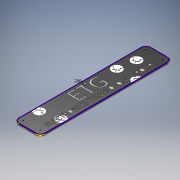
# Autodesk Inventor part: EtgSignModV5Texture2
Saved by Autodesk Inventor 2019 (Build 230136000, 136)
## iProperties
Created: 2018-10-30
Part Number: EtgSignModV5Texture2
Material: Generic
Document SubType Name: Modeling
Designer: Administrator
Density: 1 g/cm^3
Appearance: Default
Author: Administrator
Autodesk Inventor part; units mm, degrees
ref_plane "YZ Plane" through (0, 0, 0) normal (1, 0, 0) x (0, 1, 0)
ref_plane "XZ Plane" through (0, 0, 0) normal (0, 1, 0) x (-1, 0, 0)
ref_plane "XY Plane" through (0, 0, 0) normal (0, 0, 1) x (1, 0, 0)
sketch "Sketch1" plane through (0, 0, 0) normal (0, 1, 0) x (-1, 0, 0)
  line L0 (53.975, 0) -> (250.825, 0)
  line L1 (304.8, -53.975) -> (304.8, -1470.025)
  line L2 (250.825, -1524) -> (53.975, -1524)
  line L3 (0, -1470.025) -> (0, -53.975)
  circle A0 centre (263.525, -41.275) radius 5.5563
  circle A1 centre (263.525, -762) radius 5.5563
  circle A2 centre (263.525, -1482.725) radius 5.5563
  circle A3 centre (41.275, -41.275) radius 5.5563
  circle A4 centre (41.275, -762) radius 5.5563
  circle A5 centre (41.275, -1482.725) radius 5.5563
  arc A6 (304.8, -53.975) -> (250.825, 0) centre (250.825, -53.975) ccw
  arc A7 (0, -1470.025) -> (53.975, -1524) centre (53.975, -1470.025) ccw
  arc A8 (250.825, -1524) -> (304.8, -1470.025) centre (250.825, -1470.025) ccw
  arc A9 (53.975, 0) -> (0, -53.975) centre (53.975, -53.975) ccw
  point P0 (0, 0)
  point P1 (304.8, -1524)
  point P2 (0, -1524)
  dimension "d0" = 304.8
  dimension "d1" = 1524
  dimension "d2" = 11.1125
  dimension "d5" = 720.725
  dimension "d8" = 222.25
  dimension "d11" = 41.275
  dimension "d12" = 41.275
  dimension "d13" = 53.975
  constraints: 10 centre point, 8 end point, 8 point on circle, 8 tangent, 6 point on line, 3 equal radius, 2 horizontal, 2 parallel, 1 perpendicular, 1 vertical, 10 other
  measures "d0" distance of point (304.8, -1524) point (0, -1524)
  measures "d1" distance between parallel lines of L2 L0
  measures "d2" diameter of A0
  measures "d5" distance of A0.centre A1.centre
  measures "d8" distance of A0.centre A3.centre
  measures "d11" distance from line of L0 A0.centre
  measures "d12" distance from line of L1 A0.centre
  measures "d13" radius of A6
extrude "Extrusion1" add sketch "Sketch1" along normal blind 22.225
ref_plane "Work Plane3" through (0, 17.4625, 0) normal (0, 1, 0) x (1, 0, 0)
sketch "Sketch2" plane through (0, 17.4625, 0) normal (0, 1, 0) x (1, 0, 0)
  circle A0 centre (-41.275, 1482.725) radius 5.5562 projected
  circle A1 centre (-41.275, 762) radius 5.5562 projected
  circle A2 centre (-41.275, 41.275) radius 5.5562 projected
  circle A3 centre (-263.525, 1482.725) radius 5.5562 projected
  circle A4 centre (-263.525, 762) radius 5.5562 projected
  circle A5 centre (-263.525, 41.275) radius 5.5562 projected
  line L0 (-250.825, 0) -> (-53.975, 0) projected
  arc A6 (-53.975, 0) -> (0, 53.975) centre (-53.975, 53.975) ccw projected
  line L1 (0, 53.975) -> (0, 1470.025) projected
  arc A7 (0, 1470.025) -> (-53.975, 1524) centre (-53.975, 1470.025) ccw projected
  line L2 (-53.975, 1524) -> (-250.825, 1524) projected
  arc A8 (-250.825, 1524) -> (-304.8, 1470.025) centre (-250.825, 1470.025) ccw projected
  line L3 (-304.8, 1470.025) -> (-304.8, 53.975) projected
  arc A9 (-304.8, 53.975) -> (-250.825, 0) centre (-250.825, 53.975) ccw projected
  line L4 (0, 53.975) -> (0, 1470.025)
  arc A10 (-250.825, 1524) -> (-304.8, 1470.025) centre (-250.825, 1470.025) ccw projected
  line L5 (-53.975, 1524) -> (-250.825, 1524)
  line L6 (-304.8, 1470.025) -> (-304.8, 53.975) projected
  line L7 (-304.8, 1470.025) -> (-304.8, 53.975)
  line L8 (-250.825, 0) -> (-53.975, 0)
  point P0 (0, 0)
  constraints: 8 end point, 2 horizontal, 2 vertical, 1 tangent
ref_plane "Work Plane4" through (0, 4.7625, 0) normal (0, -1, 0) x (1, 0, 0)
sketch "Sketch3" plane through (0, 4.7625, 0) normal (0, -1, 0) x (1, 0, 0)
  circle A0 centre (-41.275, -1482.725) radius 5.5562 projected
  circle A1 centre (-41.275, -762) radius 5.5562 projected
  circle A2 centre (-41.275, -41.275) radius 5.5562 projected
  circle A3 centre (-263.525, -1482.725) radius 5.5562 projected
  circle A4 centre (-263.525, -762) radius 5.5562 projected
  circle A5 centre (-263.525, -41.275) radius 5.5562 projected
  line L0 (-250.825, 0) -> (-53.975, 0) projected
  arc A6 (0, -53.975) -> (-53.975, 0) centre (-53.975, -53.975) ccw projected
  line L1 (0, -53.975) -> (0, -1470.025) projected
  arc A7 (-53.975, -1524) -> (0, -1470.025) centre (-53.975, -1470.025) ccw projected
  line L2 (-53.975, -1524) -> (-250.825, -1524) projected
  arc A8 (-304.8, -1470.025) -> (-250.825, -1524) centre (-250.825, -1470.025) ccw projected
  line L3 (-304.8, -1470.025) -> (-304.8, -53.975) projected
  arc A9 (-250.825, 0) -> (-304.8, -53.975) centre (-250.825, -53.975) ccw projected
  line L4 (-299.72, -53.975) -> (-299.72, -1470.025)
  arc A10 (-299.72, -1470.025) -> (-250.825, -1518.92) centre (-250.825, -1470.025) ccw
  line L5 (-250.825, -1518.92) -> (-53.975, -1518.92)
  arc A11 (-53.975, -1518.92) -> (-5.08, -1470.025) centre (-53.975, -1470.025) ccw
  line L6 (-5.08, -1470.025) -> (-5.08, -53.975)
  arc A12 (-5.08, -53.975) -> (-53.975, -5.08) centre (-53.975, -53.975) ccw
  line L7 (-53.975, -5.08) -> (-250.825, -5.08)
  arc A13 (-250.825, -5.08) -> (-299.72, -53.975) centre (-250.825, -53.975) ccw
  point P0 (0, 0)
  dimension "d26" = 5.08
  constraints: 8 end point, 8 point on circle, 4 centre point, 7 other
  measures "d26" distance between parallel lines of L3 L4
sketch "Sketch8" plane through (0, 22.225, 0) normal (0, 1, 0) x (1, 0, 0)
  arc A0 (-53.975, 0) -> (0, 53.975) centre (-53.975, 53.975) ccw projected
  line L0 (-250.825, 0) -> (-53.975, 0) projected
  line L1 (-53.975, 0) -> (-250.825, 0)
  arc A1 (-304.8, 53.975) -> (-250.825, 0) centre (-250.825, 53.975) ccw projected
  arc A2 (-250.825, 1524) -> (-304.8, 1470.025) centre (-250.825, 1470.025) ccw projected
  line L2 (-304.8, 53.975) -> (-304.8, 1470.025)
  line L3 (-53.975, 1524) -> (-250.825, 1524) projected
  line L4 (-250.825, 1524) -> (-53.975, 1524)
  arc A3 (0, 1470.025) -> (-53.975, 1524) centre (-53.975, 1470.025) ccw projected
  line L5 (0, 1470.025) -> (0, 53.975)
  arc A4 (-53.975, 0) -> (0, 53.975) centre (-53.975, 53.975) ccw
  arc A5 (-304.8, 53.975) -> (-250.825, 0) centre (-250.825, 53.975) ccw
  arc A6 (-250.825, 1524) -> (-304.8, 1470.025) centre (-250.825, 1470.025) ccw
  arc A7 (0, 1470.025) -> (-53.975, 1524) centre (-53.975, 1470.025) ccw
  line L6 (-299.72, 1470.025) -> (-299.72, 53.975)
  arc A8 (-299.72, 53.975) -> (-250.825, 5.08) centre (-250.825, 53.975) ccw
  line L7 (-250.825, 5.08) -> (-53.975, 5.08)
  arc A9 (-53.975, 5.08) -> (-5.08, 53.975) centre (-53.975, 53.975) ccw
  line L8 (-5.08, 53.975) -> (-5.08, 1470.025)
  arc A10 (-5.08, 1470.025) -> (-53.975, 1518.92) centre (-53.975, 1470.025) ccw
  line L9 (-53.975, 1518.92) -> (-250.825, 1518.92)
  arc A11 (-250.825, 1518.92) -> (-299.72, 1470.025) centre (-250.825, 1470.025) ccw
  point P0 (0, 0)
  dimension "d25" = 5.08
  constraints: 16 end point, 16 point on circle, 9 tangent, 8 centre point, 2 horizontal, 2 vertical, 7 other
  measures "d25" distance between parallel lines of L2 L6
extrude "Extrusion2" cut sketch "Sketch3" against normal blind 12.7 contours L0 A6 L1 A7 L2 A8 L3 A9
sketch "Sketch9" plane through (0, 22.225, 0) normal (0, 1, 0) x (1, 0, 0)
  line L0 (-277.7202, 559.4153) -> (-277.7202, 933.7904) construction
  line L1 (-277.7202, 933.7904) -> (-121.9334, 933.7904) construction
  line L2 (-121.9334, 933.7904) -> (-121.9334, 559.4153) construction
  line L3 (-121.9334, 559.4153) -> (-277.7202, 559.4153) construction
  line L4 (-97.4713, 134.8938) -> (-97.4713, 1364.0426) construction
  line L5 (-97.4713, 1364.0426) -> (-40.6857, 1364.0426) construction
  line L6 (-40.6857, 1364.0426) -> (-40.6857, 134.8938) construction
  line L7 (-40.6857, 134.8938) -> (-97.4713, 134.8938) construction
  line L8 (-124.8544, 574.6289) -> (-275.0426, 574.6289)
  line L9 (-275.0426, 574.6289) -> (-275.0426, 668.5878)
  line L10 (-275.0426, 668.5878) -> (-257.2731, 668.5878)
  line L11 (-257.2731, 668.5878) -> (-257.2731, 594.5891)
  line L12 (-257.2731, 594.5891) -> (-216.1357, 594.5891)
  line L13 (-216.1357, 594.5891) -> (-216.1357, 663.5977)
  line L14 (-216.1357, 663.5977) -> (-198.3663, 663.5977)
  line L15 (-198.3663, 663.5977) -> (-198.3663, 594.5891)
  line L16 (-198.3663, 594.5891) -> (-142.6238, 594.5891)
  line L17 (-142.6238, 594.5891) -> (-142.6238, 668.5878)
  line L18 (-142.6238, 668.5878) -> (-124.8544, 668.5878)
  line L19 (-124.8544, 668.5878) -> (-124.8544, 574.6289)
  line L20 (-124.8544, 725.5473) -> (-257.2731, 725.5473)
  line L21 (-257.2731, 725.5473) -> (-257.2731, 675.16)
  line L22 (-257.2731, 675.16) -> (-275.0426, 675.16)
  line L23 (-275.0426, 675.16) -> (-275.0426, 795.8948)
  line L24 (-275.0426, 795.8948) -> (-257.2731, 795.8948)
  line L25 (-257.2731, 795.8948) -> (-257.2731, 745.5075)
  line L26 (-257.2731, 745.5075) -> (-124.8544, 745.5075)
  line L27 (-124.8544, 745.5075) -> (-124.8544, 725.5473)
  spline S0 degree 2 poles (-121.9334, 874.0316) (-121.9334, 858.0878) (-131.6701, 831.6771) (-141.5284, 822.1838) knots 0 0 0 1 2 2 2
  spline S1 degree 2 poles (-141.5284, 822.1838) (-151.5085, 812.6906) (-180.962, 802.5888) (-200.0702, 802.5888) knots 0 0 0 1 2 2 2
  spline S2 degree 2 poles (-200.0702, 802.5888) (-218.2047, 802.5888) (-246.9279, 812.8123) (-257.1514, 822.3055) knots 0 0 0 1 2 2 2
  spline S3 degree 2 poles (-257.1514, 822.3055) (-267.0098, 831.4337) (-277.7202, 858.2095) (-277.7202, 874.1533) knots 0 0 0 1 2 2 2
  spline S4 degree 2 poles (-277.7202, 874.1533) (-277.7202, 881.8209) (-275.5294, 895.6957) (-273.5821, 902.0245) knots 0 0 0 1 2 2 2
  spline S5 degree 2 poles (-273.5821, 902.0245) (-272.1216, 907.1363) (-266.7664, 919.5506) (-264.8191, 923.3235) knots 0 0 0 1 2 2 2
  line L28 (-264.8191, 923.3235) -> (-240.7208, 923.3235)
  line L29 (-240.7208, 923.3235) -> (-240.7208, 921.6196)
  spline S6 degree 2 poles (-240.7208, 921.6196) (-244.0069, 917.8466) (-249.9706, 909.9356) (-253.3785, 902.6331) knots 0 0 0 1 2 2 2
  spline S7 degree 2 poles (-253.3785, 902.6331) (-256.4212, 896.5477) (-260.4376, 880.8473) (-260.4376, 871.8409) knots 0 0 0 1 2 2 2
  spline S8 degree 2 poles (-260.4376, 871.8409) (-260.4376, 850.1768) (-227.8197, 823.4009) (-200.6787, 823.4009) knots 0 0 0 1 2 2 2
  spline S9 degree 2 poles (-200.6787, 823.4009) (-185.5869, 823.4009) (-162.9491, 830.46) (-155.1598, 837.154) knots 0 0 0 1 2 2 2
  spline S10 degree 2 poles (-155.1598, 837.154) (-147.3704, 843.6045) (-139.216, 861.8608) (-139.216, 873.3014) knots 0 0 0 1 2 2 2
  spline S11 degree 2 poles (-139.216, 873.3014) (-139.216, 881.6992) (-141.6502, 898.495) (-144.0843, 904.2153) knots 0 0 0 1 2 2 2
  line L30 (-144.0843, 904.2153) -> (-182.9093, 904.2153)
  line L31 (-182.9093, 904.2153) -> (-182.9093, 869.4067)
  line L32 (-182.9093, 869.4067) -> (-200.4353, 869.4067)
  line L33 (-200.4353, 869.4067) -> (-200.4353, 923.9321)
  line L34 (-200.4353, 923.9321) -> (-134.8345, 923.9321)
  spline S12 degree 2 poles (-134.8345, 923.9321) (-133.1306, 920.1591) (-127.8971, 907.258) (-126.3149, 901.7811) knots 0 0 0 1 2 2 2
  spline S13 degree 2 poles (-126.3149, 901.7811) (-124.1241, 894.3569) (-121.9334, 882.4295) (-121.9334, 874.0316) knots 0 0 0 1 2 2 2
  line L35 (-41.8337, 140.4134) -> (-96.3232, 140.4134)
  line L36 (-96.3232, 140.4134) -> (-96.3232, 174.5024)
  line L37 (-96.3232, 174.5024) -> (-89.8763, 174.5024)
  line L38 (-89.8763, 174.5024) -> (-89.8763, 147.6551)
  line L39 (-89.8763, 147.6551) -> (-74.9513, 147.6551)
  line L40 (-74.9513, 147.6551) -> (-74.9513, 172.692)
  line L41 (-74.9513, 172.692) -> (-68.5045, 172.692)
  line L42 (-68.5045, 172.692) -> (-68.5045, 147.6551)
  line L43 (-68.5045, 147.6551) -> (-48.2806, 147.6551)
  line L44 (-48.2806, 147.6551) -> (-48.2806, 174.5024)
  line L45 (-48.2806, 174.5024) -> (-41.8337, 174.5024)
  line L46 (-41.8337, 174.5024) -> (-41.8337, 140.4134)
  line L47 (-41.8337, 214.0228) -> (-41.8337, 182.4506)
  line L48 (-41.8337, 182.4506) -> (-96.3232, 182.4506)
  line L49 (-96.3232, 182.4506) -> (-96.3232, 189.6924)
  line L50 (-96.3232, 189.6924) -> (-48.2806, 189.6924)
  line L51 (-48.2806, 189.6924) -> (-48.2806, 214.0228)
  line L52 (-48.2806, 214.0228) -> (-41.8337, 214.0228)
  line L53 (-41.8337, 219.719) -> (-96.3232, 219.719)
  line L54 (-96.3232, 219.719) -> (-96.3232, 253.808)
  line L55 (-96.3232, 253.808) -> (-89.8763, 253.808)
  line L56 (-89.8763, 253.808) -> (-89.8763, 226.9607)
  line L57 (-89.8763, 226.9607) -> (-74.9513, 226.9607)
  line L58 (-74.9513, 226.9607) -> (-74.9513, 251.9976)
  line L59 (-74.9513, 251.9976) -> (-68.5045, 251.9976)
  line L60 (-68.5045, 251.9976) -> (-68.5045, 226.9607)
  line L61 (-68.5045, 226.9607) -> (-48.2806, 226.9607)
  line L62 (-48.2806, 226.9607) -> (-48.2806, 253.808)
  line L63 (-48.2806, 253.808) -> (-41.8337, 253.808)
  line L64 (-41.8337, 253.808) -> (-41.8337, 219.719)
  spline S14 degree 2 poles (-40.8623, 283.0399) (-40.8623, 277.741) (-44.439, 268.7772) (-48.0157, 265.5096) knots 0 0 0 1 2 2 2
  spline S15 degree 2 poles (-48.0157, 265.5096) (-51.5482, 262.242) (-62.1459, 258.6653) (-69.0343, 258.6653) knots 0 0 0 1 2 2 2
  spline S16 degree 2 poles (-69.0343, 258.6653) (-75.8786, 258.6653) (-86.0347, 262.1537) (-89.788, 265.4654) knots 0 0 0 1 2 2 2
  spline S17 degree 2 poles (-89.788, 265.4654) (-93.453, 268.733) (-97.2947, 277.6527) (-97.2947, 283.1723) knots 0 0 0 1 2 2 2
  spline S18 degree 2 poles (-97.2947, 283.1723) (-97.2947, 285.91) (-96.4999, 290.7231) (-95.8817, 292.7544) knots 0 0 0 1 2 2 2
  spline S19 degree 2 poles (-95.8817, 292.7544) (-95.3076, 294.5206) (-93.6738, 298.1856) (-92.7024, 299.9961) knots 0 0 0 1 2 2 2
  line L65 (-92.7024, 299.9961) -> (-83.9593, 299.9961)
  line L66 (-83.9593, 299.9961) -> (-83.9593, 299.422)
  spline S20 degree 2 poles (-83.9593, 299.422) (-84.8425, 298.4506) (-87.3153, 295.4479) (-88.5075, 293.2842) knots 0 0 0 1 2 2 2
  spline S21 degree 2 poles (-88.5075, 293.2842) (-89.6556, 291.2089) (-91.1127, 286.3075) (-91.1127, 283.1282) knots 0 0 0 1 2 2 2
  spline S22 degree 2 poles (-91.1127, 283.1282) (-91.1127, 279.6398) (-88.2425, 273.4137) (-85.5048, 271.0734) knots 0 0 0 1 2 2 2
  spline S23 degree 2 poles (-85.5048, 271.0734) (-82.7229, 268.7772) (-74.289, 266.2161) (-69.0343, 266.2161) knots 0 0 0 1 2 2 2
  spline S24 degree 2 poles (-69.0343, 266.2161) (-63.4264, 266.2161) (-55.3457, 268.9097) (-52.5638, 271.25) knots 0 0 0 1 2 2 2
  spline S25 degree 2 poles (-52.5638, 271.25) (-49.8703, 273.5461) (-47.1326, 279.6839) (-47.1326, 283.1282) knots 0 0 0 1 2 2 2
  spline S26 degree 2 poles (-47.1326, 283.1282) (-47.1326, 286.2633) (-48.678, 291.6063) (-49.8261, 293.6816) knots 0 0 0 1 2 2 2
  spline S27 degree 2 poles (-49.8261, 293.6816) (-50.9742, 295.6687) (-53.3587, 298.6272) (-54.1976, 299.4662) knots 0 0 0 1 2 2 2
  line L67 (-54.1976, 299.4662) -> (-54.1976, 299.9961)
  line L68 (-54.1976, 299.9961) -> (-45.5429, 299.9961)
  spline S28 degree 2 poles (-45.5429, 299.9961) (-44.7039, 298.1856) (-43.1584, 295.0063) (-42.4519, 292.7544) knots 0 0 0 1 2 2 2
  spline S29 degree 2 poles (-42.4519, 292.7544) (-41.6571, 290.3699) (-40.8623, 286.3075) (-40.8623, 283.0399) knots 0 0 0 1 2 2 2
  line L69 (-41.8337, 319.4692) -> (-89.8763, 319.4692)
  line L70 (-89.8763, 319.4692) -> (-89.8763, 301.1883)
  line L71 (-89.8763, 301.1883) -> (-96.3232, 301.1883)
  line L72 (-96.3232, 301.1883) -> (-96.3232, 344.9919)
  line L73 (-96.3232, 344.9919) -> (-89.8763, 344.9919)
  line L74 (-89.8763, 344.9919) -> (-89.8763, 326.7109)
  line L75 (-89.8763, 326.7109) -> (-41.8337, 326.7109)
  line L76 (-41.8337, 326.7109) -> (-41.8337, 319.4692)
  line L77 (-41.8337, 392.6812) -> (-41.8337, 383.2758)
  line L78 (-41.8337, 383.2758) -> (-63.5147, 366.0547)
  line L79 (-63.5147, 366.0547) -> (-63.5147, 357.7532)
  line L80 (-63.5147, 357.7532) -> (-41.8337, 357.7532)
  line L81 (-41.8337, 357.7532) -> (-41.8337, 350.5115)
  line L82 (-41.8337, 350.5115) -> (-96.3232, 350.5115)
  line L83 (-96.3232, 350.5115) -> (-96.3232, 364.5533)
  spline S30 degree 2 poles (-96.3232, 364.5533) (-96.3232, 369.2339) (-95.3076, 375.5484) (-93.453, 378.4186) knots 0 0 0 1 2 2 2
  spline S31 degree 2 poles (-93.453, 378.4186) (-91.5985, 381.2888) (-85.8139, 384.6005) (-81.5307, 384.6005) knots 0 0 0 1 2 2 2
  spline S32 degree 2 poles (-81.5307, 384.6005) (-75.5695, 384.6005) (-67.4888, 378.5069) (-65.5459, 373.2964) knots 0 0 0 1 2 2 2
  line L84 (-65.5459, 373.2964) -> (-41.8337, 392.6812)
  spline S33 degree 2 poles (-80.9567, 377.0497) (-83.3411, 377.0497) (-87.0062, 375.3717) (-88.1984, 373.6055) knots 0 0 0 1 2 2 2
  spline S34 degree 2 poles (-88.1984, 373.6055) (-89.214, 372.06) (-90.053, 367.9534) (-90.053, 364.9507) knots 0 0 0 1 2 2 2
  line L85 (-90.053, 364.9507) -> (-90.053, 357.7532)
  line L86 (-90.053, 357.7532) -> (-69.5642, 357.7532)
  line L87 (-69.5642, 357.7532) -> (-69.5642, 364.1118)
  spline S35 degree 2 poles (-69.5642, 364.1118) (-69.5642, 367.2469) (-70.6681, 372.2366) (-72.3903, 373.9587) knots 0 0 0 1 2 2 2
  spline S36 degree 2 poles (-72.3903, 373.9587) (-73.8916, 375.5484) (-78.1306, 377.0497) (-80.9567, 377.0497) knots 0 0 0 1 2 2 2
  spline S37 degree 2 poles (-90.0971, 435.5575) (-86.4763, 438.6484) (-75.8786, 442.0927) (-69.0785, 442.0927) knots 0 0 0 1 2 2 2
  spline S38 degree 2 poles (-69.0785, 442.0927) (-62.455, 442.0927) (-51.7249, 438.7368) (-48.104, 435.5575) knots 0 0 0 1 2 2 2
  spline S39 degree 2 poles (-48.104, 435.5575) (-44.3065, 432.2016) (-40.6857, 423.326) (-40.6857, 417.9831) knots 0 0 0 1 2 2 2
  spline S40 degree 2 poles (-40.6857, 417.9831) (-40.6857, 412.4635) (-44.439, 403.6321) (-48.104, 400.4087) knots 0 0 0 1 2 2 2
  spline S41 degree 2 poles (-48.104, 400.4087) (-51.7249, 397.2735) (-62.3667, 393.9176) (-69.0785, 393.9176) knots 0 0 0 1 2 2 2
  spline S42 degree 2 poles (-69.0785, 393.9176) (-75.9228, 393.9176) (-86.3438, 397.3177) (-90.0971, 400.4528) knots 0 0 0 1 2 2 2
  spline S43 degree 2 poles (-90.0971, 400.4528) (-93.718, 403.6321) (-97.4713, 412.5076) (-97.4713, 417.9831) knots 0 0 0 1 2 2 2
  spline S44 degree 2 poles (-97.4713, 417.9831) (-97.4713, 423.5468) (-93.5855, 432.4665) (-90.0971, 435.5575) knots 0 0 0 1 2 2 2
  spline S45 degree 2 poles (-69.0785, 434.5419) (-74.4656, 434.5419) (-82.8113, 432.2016) (-85.549, 430.082) knots 0 0 0 1 2 2 2
  spline S46 degree 2 poles (-85.549, 430.082) (-88.375, 427.9183) (-91.2011, 421.8247) (-91.2011, 418.0272) knots 0 0 0 1 2 2 2
  spline S47 degree 2 poles (-91.2011, 418.0272) (-91.2011, 414.0973) (-88.4633, 408.1803) (-85.549, 405.9283) knots 0 0 0 1 2 2 2
  spline S48 degree 2 poles (-85.549, 405.9283) (-82.7671, 403.7646) (-74.3773, 401.4684) (-69.0785, 401.4684) knots 0 0 0 1 2 2 2
  spline S49 degree 2 poles (-69.0785, 401.4684) (-58.3484, 401.4684) (-46.9559, 410.4764) (-46.9559, 418.0272) knots 0 0 0 1 2 2 2
  spline S50 degree 2 poles (-46.9559, 418.0272) (-46.9559, 425.578) (-58.3484, 434.5419) (-69.0785, 434.5419) knots 0 0 0 1 2 2 2
  line L88 (-41.8337, 489.0314) -> (-41.8337, 480.9065)
  line L89 (-41.8337, 480.9065) -> (-88.8166, 456.7969)
  line L90 (-88.8166, 456.7969) -> (-41.8337, 456.7969)
  line L91 (-41.8337, 456.7969) -> (-41.8337, 450.0409)
  line L92 (-41.8337, 450.0409) -> (-96.3232, 450.0409)
  line L93 (-96.3232, 450.0409) -> (-96.3232, 460.3294)
  line L94 (-96.3232, 460.3294) -> (-53.182, 482.2754)
  line L95 (-53.182, 482.2754) -> (-96.3232, 482.2754)
  line L96 (-96.3232, 482.2754) -> (-96.3232, 489.0314)
  line L97 (-96.3232, 489.0314) -> (-41.8337, 489.0314)
  line L98 (-41.8337, 519.058) -> (-41.8337, 497.951)
  line L99 (-41.8337, 497.951) -> (-47.3975, 497.951)
  line L100 (-47.3975, 497.951) -> (-47.3975, 504.8837)
  line L101 (-47.3975, 504.8837) -> (-90.7595, 504.8837)
  line L102 (-90.7595, 504.8837) -> (-90.7595, 497.951)
  line L103 (-90.7595, 497.951) -> (-96.3232, 497.951)
  line L104 (-96.3232, 497.951) -> (-96.3232, 519.058)
  line L105 (-96.3232, 519.058) -> (-90.7595, 519.058)
  line L106 (-90.7595, 519.058) -> (-90.7595, 512.1254)
  line L107 (-90.7595, 512.1254) -> (-47.3975, 512.1254)
  line L108 (-47.3975, 512.1254) -> (-47.3975, 519.058)
  line L109 (-47.3975, 519.058) -> (-41.8337, 519.058)
  spline S51 degree 2 poles (-40.8623, 549.3054) (-40.8623, 544.0066) (-44.439, 535.0428) (-48.0157, 531.7752) knots 0 0 0 1 2 2 2
  spline S52 degree 2 poles (-48.0157, 531.7752) (-51.5482, 528.5076) (-62.1459, 524.9309) (-69.0343, 524.9309) knots 0 0 0 1 2 2 2
  spline S53 degree 2 poles (-69.0343, 524.9309) (-75.8786, 524.9309) (-86.0347, 528.4192) (-89.788, 531.731) knots 0 0 0 1 2 2 2
  spline S54 degree 2 poles (-89.788, 531.731) (-93.453, 534.9986) (-97.2947, 543.9183) (-97.2947, 549.4379) knots 0 0 0 1 2 2 2
  spline S55 degree 2 poles (-97.2947, 549.4379) (-97.2947, 552.1756) (-96.4999, 556.9887) (-95.8817, 559.0199) knots 0 0 0 1 2 2 2
  spline S56 degree 2 poles (-95.8817, 559.0199) (-95.3076, 560.7862) (-93.6738, 564.4512) (-92.7024, 566.2616) knots 0 0 0 1 2 2 2
  line L110 (-92.7024, 566.2616) -> (-83.9593, 566.2616)
  line L111 (-83.9593, 566.2616) -> (-83.9593, 565.6876)
  spline S57 degree 2 poles (-83.9593, 565.6876) (-84.8425, 564.7161) (-87.3153, 561.7135) (-88.5075, 559.5498) knots 0 0 0 1 2 2 2
  spline S58 degree 2 poles (-88.5075, 559.5498) (-89.6556, 557.4744) (-91.1127, 552.573) (-91.1127, 549.3937) knots 0 0 0 1 2 2 2
  spline S59 degree 2 poles (-91.1127, 549.3937) (-91.1127, 545.9053) (-88.2425, 539.6792) (-85.5048, 537.3389) knots 0 0 0 1 2 2 2
  spline S60 degree 2 poles (-85.5048, 537.3389) (-82.7229, 535.0428) (-74.289, 532.4817) (-69.0343, 532.4817) knots 0 0 0 1 2 2 2
  spline S61 degree 2 poles (-69.0343, 532.4817) (-63.4264, 532.4817) (-55.3457, 535.1752) (-52.5638, 537.5155) knots 0 0 0 1 2 2 2
  spline S62 degree 2 poles (-52.5638, 537.5155) (-49.8703, 539.8117) (-47.1326, 545.9495) (-47.1326, 549.3937) knots 0 0 0 1 2 2 2
  spline S63 degree 2 poles (-47.1326, 549.3937) (-47.1326, 552.5289) (-48.678, 557.8718) (-49.8261, 559.9472) knots 0 0 0 1 2 2 2
  spline S64 degree 2 poles (-49.8261, 559.9472) (-50.9742, 561.9343) (-53.3587, 564.8928) (-54.1976, 565.7317) knots 0 0 0 1 2 2 2
  line L112 (-54.1976, 565.7317) -> (-54.1976, 566.2616)
  line L113 (-54.1976, 566.2616) -> (-45.5429, 566.2616)
  spline S65 degree 2 poles (-45.5429, 566.2616) (-44.7039, 564.4512) (-43.1584, 561.2719) (-42.4519, 559.0199) knots 0 0 0 1 2 2 2
  spline S66 degree 2 poles (-42.4519, 559.0199) (-41.6571, 556.6354) (-40.8623, 552.573) (-40.8623, 549.3054) knots 0 0 0 1 2 2 2
  spline S67 degree 2 poles (-40.8623, 588.2076) (-40.8623, 582.2906) (-43.3351, 573.9891) (-45.1013, 570.3241) knots 0 0 0 1 2 2 2
  line L114 (-45.1013, 570.3241) -> (-54.1976, 570.3241)
  line L115 (-54.1976, 570.3241) -> (-54.1976, 570.8539)
  spline S68 degree 2 poles (-54.1976, 570.8539) (-50.8417, 574.4306) (-47.1326, 583.4828) (-47.1326, 587.6777) knots 0 0 0 1 2 2 2
  spline S69 degree 2 poles (-47.1326, 587.6777) (-47.1326, 593.683) (-52.1223, 599.8208) (-56.2289, 599.8208) knots 0 0 0 1 2 2 2
  spline S70 degree 2 poles (-56.2289, 599.8208) (-59.4965, 599.8208) (-63.5589, 596.5974) (-64.5745, 593.109) knots 0 0 0 1 2 2 2
  spline S71 degree 2 poles (-64.5745, 593.109) (-65.281, 590.592) (-66.2525, 586.3971) (-67.0473, 583.262) knots 0 0 0 1 2 2 2
  spline S72 degree 2 poles (-67.0473, 583.262) (-67.7979, 580.436) (-70.0499, 575.9761) (-71.8604, 574.254) knots 0 0 0 1 2 2 2
  spline S73 degree 2 poles (-71.8604, 574.254) (-73.6708, 572.5761) (-78.528, 570.7215) (-81.7073, 570.7215) knots 0 0 0 1 2 2 2
  spline S74 degree 2 poles (-81.7073, 570.7215) (-88.3309, 570.7215) (-97.2947, 581.0542) (-97.2947, 589.0465) knots 0 0 0 1 2 2 2
  spline S75 degree 2 poles (-97.2947, 589.0465) (-97.2947, 593.6389) (-95.4843, 601.7637) (-93.7621, 605.2521) knots 0 0 0 1 2 2 2
  line L116 (-93.7621, 605.2521) -> (-85.1074, 605.2521)
  line L117 (-85.1074, 605.2521) -> (-85.1074, 604.7222)
  spline S76 degree 2 poles (-85.1074, 604.7222) (-87.4919, 602.117) (-91.0244, 593.9921) (-91.0244, 589.5323) knots 0 0 0 1 2 2 2
  spline S77 degree 2 poles (-91.0244, 589.5323) (-91.0244, 584.4984) (-86.2996, 578.2723) (-82.458, 578.2723) knots 0 0 0 1 2 2 2
  spline S78 degree 2 poles (-82.458, 578.2723) (-79.0138, 578.2723) (-74.9072, 581.9373) (-73.9799, 585.3815) knots 0 0 0 1 2 2 2
  spline S79 degree 2 poles (-73.9799, 585.3815) (-73.3617, 587.6777) (-71.7721, 594.3454) (-71.1097, 596.5532) knots 0 0 0 1 2 2 2
  spline S80 degree 2 poles (-71.1097, 596.5532) (-69.3876, 602.1611) (-62.455, 607.3716) (-57.3769, 607.3716) knots 0 0 0 1 2 2 2
  spline S81 degree 2 poles (-57.3769, 607.3716) (-54.1535, 607.3716) (-47.9715, 604.7664) (-45.8079, 602.4261) knots 0 0 0 1 2 2 2
  spline S82 degree 2 poles (-45.8079, 602.4261) (-43.4234, 599.8208) (-40.8623, 593.1973) (-40.8623, 588.2076) knots 0 0 0 1 2 2 2
  line L118 (-41.8337, 650.8661) -> (-89.8763, 650.8661)
  line L119 (-89.8763, 650.8661) -> (-89.8763, 632.5852)
  line L120 (-89.8763, 632.5852) -> (-96.3232, 632.5852)
  line L121 (-96.3232, 632.5852) -> (-96.3232, 676.3887)
  line L122 (-96.3232, 676.3887) -> (-89.8763, 676.3887)
  line L123 (-89.8763, 676.3887) -> (-89.8763, 658.1078)
  line L124 (-89.8763, 658.1078) -> (-41.8337, 658.1078)
  line L125 (-41.8337, 658.1078) -> (-41.8337, 650.8661)
  line L126 (-41.8337, 681.9083) -> (-96.3232, 681.9083)
  line L127 (-96.3232, 681.9083) -> (-96.3232, 715.9974)
  line L128 (-96.3232, 715.9974) -> (-89.8763, 715.9974)
  line L129 (-89.8763, 715.9974) -> (-89.8763, 689.15)
  line L130 (-89.8763, 689.15) -> (-74.9513, 689.15)
  line L131 (-74.9513, 689.15) -> (-74.9513, 714.1869)
  line L132 (-74.9513, 714.1869) -> (-68.5045, 714.1869)
  line L133 (-68.5045, 714.1869) -> (-68.5045, 689.15)
  line L134 (-68.5045, 689.15) -> (-48.2806, 689.15)
  line L135 (-48.2806, 689.15) -> (-48.2806, 715.9974)
  line L136 (-48.2806, 715.9974) -> (-41.8337, 715.9974)
  line L137 (-41.8337, 715.9974) -> (-41.8337, 681.9083)
  spline S83 degree 2 poles (-40.8623, 745.2292) (-40.8623, 739.9304) (-44.439, 730.9665) (-48.0157, 727.6989) knots 0 0 0 1 2 2 2
  spline S84 degree 2 poles (-48.0157, 727.6989) (-51.5482, 724.4313) (-62.1459, 720.8546) (-69.0343, 720.8546) knots 0 0 0 1 2 2 2
  spline S85 degree 2 poles (-69.0343, 720.8546) (-75.8786, 720.8546) (-86.0347, 724.343) (-89.788, 727.6548) knots 0 0 0 1 2 2 2
  spline S86 degree 2 poles (-89.788, 727.6548) (-93.453, 730.9224) (-97.2947, 739.842) (-97.2947, 745.3616) knots 0 0 0 1 2 2 2
  spline S87 degree 2 poles (-97.2947, 745.3616) (-97.2947, 748.0994) (-96.4999, 752.9125) (-95.8817, 754.9437) knots 0 0 0 1 2 2 2
  spline S88 degree 2 poles (-95.8817, 754.9437) (-95.3076, 756.7099) (-93.6738, 760.375) (-92.7024, 762.1854) knots 0 0 0 1 2 2 2
  line L138 (-92.7024, 762.1854) -> (-83.9593, 762.1854)
  line L139 (-83.9593, 762.1854) -> (-83.9593, 761.6114)
  spline S89 degree 2 poles (-83.9593, 761.6114) (-84.8425, 760.6399) (-87.3153, 757.6372) (-88.5075, 755.4736) knots 0 0 0 1 2 2 2
  spline S90 degree 2 poles (-88.5075, 755.4736) (-89.6556, 753.3982) (-91.1127, 748.4968) (-91.1127, 745.3175) knots 0 0 0 1 2 2 2
  spline S91 degree 2 poles (-91.1127, 745.3175) (-91.1127, 741.8291) (-88.2425, 735.603) (-85.5048, 733.2627) knots 0 0 0 1 2 2 2
  spline S92 degree 2 poles (-85.5048, 733.2627) (-82.7229, 730.9665) (-74.289, 728.4054) (-69.0343, 728.4054) knots 0 0 0 1 2 2 2
  spline S93 degree 2 poles (-69.0343, 728.4054) (-63.4264, 728.4054) (-55.3457, 731.099) (-52.5638, 733.4393) knots 0 0 0 1 2 2 2
  spline S94 degree 2 poles (-52.5638, 733.4393) (-49.8703, 735.7355) (-47.1326, 741.8733) (-47.1326, 745.3175) knots 0 0 0 1 2 2 2
  spline S95 degree 2 poles (-47.1326, 745.3175) (-47.1326, 748.4526) (-48.678, 753.7956) (-49.8261, 755.871) knots 0 0 0 1 2 2 2
  spline S96 degree 2 poles (-49.8261, 755.871) (-50.9742, 757.858) (-53.3587, 760.8165) (-54.1976, 761.6555) knots 0 0 0 1 2 2 2
  line L140 (-54.1976, 761.6555) -> (-54.1976, 762.1854)
  line L141 (-54.1976, 762.1854) -> (-45.5429, 762.1854)
  spline S97 degree 2 poles (-45.5429, 762.1854) (-44.7039, 760.375) (-43.1584, 757.1957) (-42.4519, 754.9437) knots 0 0 0 1 2 2 2
  spline S98 degree 2 poles (-42.4519, 754.9437) (-41.6571, 752.5592) (-40.8623, 748.4968) (-40.8623, 745.2292) knots 0 0 0 1 2 2 2
  line L142 (-41.8337, 808.5059) -> (-41.8337, 801.2642)
  line L143 (-41.8337, 801.2642) -> (-68.5045, 801.2642)
  line L144 (-68.5045, 801.2642) -> (-68.5045, 776.1831)
  line L145 (-68.5045, 776.1831) -> (-41.8337, 776.1831)
  line L146 (-41.8337, 776.1831) -> (-41.8337, 768.9414)
  line L147 (-41.8337, 768.9414) -> (-96.3232, 768.9414)
  line L148 (-96.3232, 768.9414) -> (-96.3232, 776.1831)
  line L149 (-96.3232, 776.1831) -> (-74.9513, 776.1831)
  line L150 (-74.9513, 776.1831) -> (-74.9513, 801.2642)
  line L151 (-74.9513, 801.2642) -> (-96.3232, 801.2642)
  line L152 (-96.3232, 801.2642) -> (-96.3232, 808.5059)
  line L153 (-96.3232, 808.5059) -> (-41.8337, 808.5059)
  line L154 (-41.8337, 858.5356) -> (-41.8337, 850.4107)
  line L155 (-41.8337, 850.4107) -> (-88.8166, 826.3011)
  line L156 (-88.8166, 826.3011) -> (-41.8337, 826.3011)
  line L157 (-41.8337, 826.3011) -> (-41.8337, 819.5451)
  line L158 (-41.8337, 819.5451) -> (-96.3232, 819.5451)
  line L159 (-96.3232, 819.5451) -> (-96.3232, 829.8336)
  line L160 (-96.3232, 829.8336) -> (-53.182, 851.7796)
  line L161 (-53.182, 851.7796) -> (-96.3232, 851.7796)
  line L162 (-96.3232, 851.7796) -> (-96.3232, 858.5356)
  line L163 (-96.3232, 858.5356) -> (-41.8337, 858.5356)
  spline S99 degree 2 poles (-90.0971, 908.1236) (-86.4763, 911.2146) (-75.8786, 914.6589) (-69.0785, 914.6589) knots 0 0 0 1 2 2 2
  spline S100 degree 2 poles (-69.0785, 914.6589) (-62.455, 914.6589) (-51.7249, 911.3029) (-48.104, 908.1236) knots 0 0 0 1 2 2 2
  spline S101 degree 2 poles (-48.104, 908.1236) (-44.3065, 904.7677) (-40.6857, 895.8922) (-40.6857, 890.5492) knots 0 0 0 1 2 2 2
  spline S102 degree 2 poles (-40.6857, 890.5492) (-40.6857, 885.0296) (-44.439, 876.1983) (-48.104, 872.9748) knots 0 0 0 1 2 2 2
  spline S103 degree 2 poles (-48.104, 872.9748) (-51.7249, 869.8397) (-62.3667, 866.4838) (-69.0785, 866.4838) knots 0 0 0 1 2 2 2
  spline S104 degree 2 poles (-69.0785, 866.4838) (-75.9228, 866.4838) (-86.3438, 869.8839) (-90.0971, 873.019) knots 0 0 0 1 2 2 2
  spline S105 degree 2 poles (-90.0971, 873.019) (-93.718, 876.1983) (-97.4713, 885.0738) (-97.4713, 890.5492) knots 0 0 0 1 2 2 2
  spline S106 degree 2 poles (-97.4713, 890.5492) (-97.4713, 896.113) (-93.5855, 905.0327) (-90.0971, 908.1236) knots 0 0 0 1 2 2 2
  spline S107 degree 2 poles (-69.0785, 907.108) (-74.4656, 907.108) (-82.8113, 904.7677) (-85.549, 902.6482) knots 0 0 0 1 2 2 2
  spline S108 degree 2 poles (-85.549, 902.6482) (-88.375, 900.4845) (-91.2011, 894.3909) (-91.2011, 890.5934) knots 0 0 0 1 2 2 2
  spline S109 degree 2 poles (-91.2011, 890.5934) (-91.2011, 886.6634) (-88.4633, 880.7464) (-85.549, 878.4944) knots 0 0 0 1 2 2 2
  spline S110 degree 2 poles (-85.549, 878.4944) (-82.7671, 876.3307) (-74.3773, 874.0346) (-69.0785, 874.0346) knots 0 0 0 1 2 2 2
  spline S111 degree 2 poles (-69.0785, 874.0346) (-58.3484, 874.0346) (-46.9559, 883.0426) (-46.9559, 890.5934) knots 0 0 0 1 2 2 2
  spline S112 degree 2 poles (-46.9559, 890.5934) (-46.9559, 898.1442) (-58.3484, 907.108) (-69.0785, 907.108) knots 0 0 0 1 2 2 2
  line L164 (-41.8337, 954.1792) -> (-41.8337, 922.6071)
  line L165 (-41.8337, 922.6071) -> (-96.3232, 922.6071)
  line L166 (-96.3232, 922.6071) -> (-96.3232, 929.8488)
  line L167 (-96.3232, 929.8488) -> (-48.2806, 929.8488)
  line L168 (-48.2806, 929.8488) -> (-48.2806, 954.1792)
  line L169 (-48.2806, 954.1792) -> (-41.8337, 954.1792)
  spline S113 degree 2 poles (-90.0971, 998.4243) (-86.4763, 1001.5153) (-75.8786, 1004.9595) (-69.0785, 1004.9595) knots 0 0 0 1 2 2 2
  spline S114 degree 2 poles (-69.0785, 1004.9595) (-62.455, 1004.9595) (-51.7249, 1001.6036) (-48.104, 998.4243) knots 0 0 0 1 2 2 2
  spline S115 degree 2 poles (-48.104, 998.4243) (-44.3065, 995.0684) (-40.6857, 986.1929) (-40.6857, 980.8499) knots 0 0 0 1 2 2 2
  spline S116 degree 2 poles (-40.6857, 980.8499) (-40.6857, 975.3303) (-44.439, 966.499) (-48.104, 963.2755) knots 0 0 0 1 2 2 2
  spline S117 degree 2 poles (-48.104, 963.2755) (-51.7249, 960.1404) (-62.3667, 956.7845) (-69.0785, 956.7845) knots 0 0 0 1 2 2 2
  spline S118 degree 2 poles (-69.0785, 956.7845) (-75.9228, 956.7845) (-86.3438, 960.1845) (-90.0971, 963.3197) knots 0 0 0 1 2 2 2
  spline S119 degree 2 poles (-90.0971, 963.3197) (-93.718, 966.499) (-97.4713, 975.3745) (-97.4713, 980.8499) knots 0 0 0 1 2 2 2
  spline S120 degree 2 poles (-97.4713, 980.8499) (-97.4713, 986.4137) (-93.5855, 995.3333) (-90.0971, 998.4243) knots 0 0 0 1 2 2 2
  spline S121 degree 2 poles (-69.0785, 997.4087) (-74.4656, 997.4087) (-82.8113, 995.0684) (-85.549, 992.9489) knots 0 0 0 1 2 2 2
  spline S122 degree 2 poles (-85.549, 992.9489) (-88.375, 990.7852) (-91.2011, 984.6916) (-91.2011, 980.8941) knots 0 0 0 1 2 2 2
  spline S123 degree 2 poles (-91.2011, 980.8941) (-91.2011, 976.9641) (-88.4633, 971.0471) (-85.549, 968.7951) knots 0 0 0 1 2 2 2
  spline S124 degree 2 poles (-85.549, 968.7951) (-82.7671, 966.6314) (-74.3773, 964.3353) (-69.0785, 964.3353) knots 0 0 0 1 2 2 2
  spline S125 degree 2 poles (-69.0785, 964.3353) (-58.3484, 964.3353) (-46.9559, 973.3433) (-46.9559, 980.8941) knots 0 0 0 1 2 2 2
  spline S126 degree 2 poles (-46.9559, 980.8941) (-46.9559, 988.4449) (-58.3484, 997.4087) (-69.0785, 997.4087) knots 0 0 0 1 2 2 2
  spline S127 degree 2 poles (-40.774, 1035.7368) (-40.774, 1029.9523) (-44.3065, 1020.3703) (-47.8832, 1016.926) knots 0 0 0 1 2 2 2
  spline S128 degree 2 poles (-47.8832, 1016.926) (-51.5041, 1013.4818) (-62.19, 1009.8168) (-69.1226, 1009.8168) knots 0 0 0 1 2 2 2
  spline S129 degree 2 poles (-69.1226, 1009.8168) (-75.702, 1009.8168) (-86.123, 1013.526) (-89.8322, 1016.9702) knots 0 0 0 1 2 2 2
  spline S130 degree 2 poles (-89.8322, 1016.9702) (-93.4089, 1020.2819) (-97.2947, 1029.9964) (-97.2947, 1035.781) knots 0 0 0 1 2 2 2
  spline S131 degree 2 poles (-97.2947, 1035.781) (-97.2947, 1038.5629) (-96.4999, 1043.5967) (-95.7934, 1045.8929) knots 0 0 0 1 2 2 2
  spline S132 degree 2 poles (-95.7934, 1045.8929) (-95.2635, 1047.7475) (-93.3206, 1052.2515) (-92.6141, 1053.6203) knots 0 0 0 1 2 2 2
  line L170 (-92.6141, 1053.6203) -> (-83.871, 1053.6203)
  line L171 (-83.871, 1053.6203) -> (-83.871, 1053.0021)
  spline S133 degree 2 poles (-83.871, 1053.0021) (-85.0633, 1051.6333) (-87.2269, 1048.7631) (-88.4633, 1046.1137) knots 0 0 0 1 2 2 2
  spline S134 degree 2 poles (-88.4633, 1046.1137) (-89.5673, 1043.9058) (-91.0244, 1038.2096) (-91.0244, 1034.942) knots 0 0 0 1 2 2 2
  spline S135 degree 2 poles (-91.0244, 1034.942) (-91.0244, 1027.0821) (-79.1904, 1017.3676) (-69.3434, 1017.3676) knots 0 0 0 1 2 2 2
  spline S136 degree 2 poles (-69.3434, 1017.3676) (-63.868, 1017.3676) (-55.6548, 1019.9287) (-52.8288, 1022.3573) knots 0 0 0 1 2 2 2
  spline S137 degree 2 poles (-52.8288, 1022.3573) (-50.0027, 1024.6976) (-47.0442, 1031.3211) (-47.0442, 1035.4719) knots 0 0 0 1 2 2 2
  spline S138 degree 2 poles (-47.0442, 1035.4719) (-47.0442, 1038.5187) (-47.9274, 1044.6123) (-48.8105, 1046.6877) knots 0 0 0 1 2 2 2
  line L172 (-48.8105, 1046.6877) -> (-62.8965, 1046.6877)
  line L173 (-62.8965, 1046.6877) -> (-62.8965, 1034.0589)
  line L174 (-62.8965, 1034.0589) -> (-69.2551, 1034.0589)
  line L175 (-69.2551, 1034.0589) -> (-69.2551, 1053.8411)
  line L176 (-69.2551, 1053.8411) -> (-45.4546, 1053.8411)
  spline S139 degree 2 poles (-45.4546, 1053.8411) (-44.8364, 1052.4723) (-42.9377, 1047.7916) (-42.3636, 1045.8046) knots 0 0 0 1 2 2 2
  spline S140 degree 2 poles (-42.3636, 1045.8046) (-41.5688, 1043.111) (-40.774, 1038.7836) (-40.774, 1035.7368) knots 0 0 0 1 2 2 2
  line L177 (-96.3232, 1101.0889) -> (-65.9434, 1082.6755)
  line L178 (-65.9434, 1082.6755) -> (-41.8337, 1082.6755)
  line L179 (-41.8337, 1082.6755) -> (-41.8337, 1075.4338)
  line L180 (-41.8337, 1075.4338) -> (-65.1927, 1075.4338)
  line L181 (-65.1927, 1075.4338) -> (-96.3232, 1057.0204)
  line L182 (-96.3232, 1057.0204) -> (-96.3232, 1065.0569)
  line L183 (-96.3232, 1065.0569) -> (-72.3461, 1079.0988)
  line L184 (-72.3461, 1079.0988) -> (-96.3232, 1093.4056)
  line L185 (-96.3232, 1093.4056) -> (-96.3232, 1101.0889)
  spline S141 degree 2 poles (-40.774, 1152.355) (-40.774, 1146.5704) (-44.3065, 1136.9884) (-47.8832, 1133.5442) knots 0 0 0 1 2 2 2
  spline S142 degree 2 poles (-47.8832, 1133.5442) (-51.5041, 1130.0999) (-62.19, 1126.4349) (-69.1226, 1126.4349) knots 0 0 0 1 2 2 2
  spline S143 degree 2 poles (-69.1226, 1126.4349) (-75.702, 1126.4349) (-86.123, 1130.1441) (-89.8322, 1133.5883) knots 0 0 0 1 2 2 2
  spline S144 degree 2 poles (-89.8322, 1133.5883) (-93.4089, 1136.9001) (-97.2947, 1146.6146) (-97.2947, 1152.3991) knots 0 0 0 1 2 2 2
  spline S145 degree 2 poles (-97.2947, 1152.3991) (-97.2947, 1155.181) (-96.4999, 1160.2149) (-95.7934, 1162.511) knots 0 0 0 1 2 2 2
  spline S146 degree 2 poles (-95.7934, 1162.511) (-95.2635, 1164.3656) (-93.3206, 1168.8696) (-92.6141, 1170.2385) knots 0 0 0 1 2 2 2
  line L186 (-92.6141, 1170.2385) -> (-83.871, 1170.2385)
  line L187 (-83.871, 1170.2385) -> (-83.871, 1169.6203)
  spline S147 degree 2 poles (-83.871, 1169.6203) (-85.0633, 1168.2514) (-87.2269, 1165.3812) (-88.4633, 1162.7318) knots 0 0 0 1 2 2 2
  spline S148 degree 2 poles (-88.4633, 1162.7318) (-89.5673, 1160.524) (-91.0244, 1154.8277) (-91.0244, 1151.5601) knots 0 0 0 1 2 2 2
  spline S149 degree 2 poles (-91.0244, 1151.5601) (-91.0244, 1143.7002) (-79.1904, 1133.9857) (-69.3434, 1133.9857) knots 0 0 0 1 2 2 2
  spline S150 degree 2 poles (-69.3434, 1133.9857) (-63.868, 1133.9857) (-55.6548, 1136.5468) (-52.8288, 1138.9754) knots 0 0 0 1 2 2 2
  spline S151 degree 2 poles (-52.8288, 1138.9754) (-50.0027, 1141.3158) (-47.0442, 1147.9393) (-47.0442, 1152.09) knots 0 0 0 1 2 2 2
  spline S152 degree 2 poles (-47.0442, 1152.09) (-47.0442, 1155.1368) (-47.9274, 1161.2305) (-48.8105, 1163.3059) knots 0 0 0 1 2 2 2
  line L188 (-48.8105, 1163.3059) -> (-62.8965, 1163.3059)
  line L189 (-62.8965, 1163.3059) -> (-62.8965, 1150.677)
  line L190 (-62.8965, 1150.677) -> (-69.2551, 1150.677)
  line L191 (-69.2551, 1150.677) -> (-69.2551, 1170.4593)
  line L192 (-69.2551, 1170.4593) -> (-45.4546, 1170.4593)
  spline S153 degree 2 poles (-45.4546, 1170.4593) (-44.8364, 1169.0904) (-42.9377, 1164.4098) (-42.3636, 1162.4227) knots 0 0 0 1 2 2 2
  spline S154 degree 2 poles (-42.3636, 1162.4227) (-41.5688, 1159.7291) (-40.774, 1155.4018) (-40.774, 1152.355) knots 0 0 0 1 2 2 2
  line L193 (-41.8337, 1221.7253) -> (-41.8337, 1212.3199)
  line L194 (-41.8337, 1212.3199) -> (-63.5147, 1195.0988)
  line L195 (-63.5147, 1195.0988) -> (-63.5147, 1186.7973)
  line L196 (-63.5147, 1186.7973) -> (-41.8337, 1186.7973)
  line L197 (-41.8337, 1186.7973) -> (-41.8337, 1179.5556)
  line L198 (-41.8337, 1179.5556) -> (-96.3232, 1179.5556)
  line L199 (-96.3232, 1179.5556) -> (-96.3232, 1193.5974)
  spline S155 degree 2 poles (-96.3232, 1193.5974) (-96.3232, 1198.278) (-95.3076, 1204.5925) (-93.453, 1207.4627) knots 0 0 0 1 2 2 2
  spline S156 degree 2 poles (-93.453, 1207.4627) (-91.5985, 1210.3329) (-85.8139, 1213.6446) (-81.5307, 1213.6446) knots 0 0 0 1 2 2 2
  spline S157 degree 2 poles (-81.5307, 1213.6446) (-75.5695, 1213.6446) (-67.4888, 1207.551) (-65.5459, 1202.3405) knots 0 0 0 1 2 2 2
  line L200 (-65.5459, 1202.3405) -> (-41.8337, 1221.7253)
  spline S158 degree 2 poles (-80.9567, 1206.0938) (-83.3411, 1206.0938) (-87.0062, 1204.4158) (-88.1984, 1202.6496) knots 0 0 0 1 2 2 2
  spline S159 degree 2 poles (-88.1984, 1202.6496) (-89.214, 1201.1041) (-90.053, 1196.9975) (-90.053, 1193.9948) knots 0 0 0 1 2 2 2
  line L201 (-90.053, 1193.9948) -> (-90.053, 1186.7973)
  line L202 (-90.053, 1186.7973) -> (-69.5642, 1186.7973)
  line L203 (-69.5642, 1186.7973) -> (-69.5642, 1193.1559)
  spline S160 degree 2 poles (-69.5642, 1193.1559) (-69.5642, 1196.291) (-70.6681, 1201.2807) (-72.3903, 1203.0028) knots 0 0 0 1 2 2 2
  spline S161 degree 2 poles (-72.3903, 1203.0028) (-73.8916, 1204.5925) (-78.1306, 1206.0938) (-80.9567, 1206.0938) knots 0 0 0 1 2 2 2
  spline S162 degree 2 poles (-90.0971, 1264.6016) (-86.4763, 1267.6925) (-75.8786, 1271.1368) (-69.0785, 1271.1368) knots 0 0 0 1 2 2 2
  spline S163 degree 2 poles (-69.0785, 1271.1368) (-62.455, 1271.1368) (-51.7249, 1267.7809) (-48.104, 1264.6016) knots 0 0 0 1 2 2 2
  spline S164 degree 2 poles (-48.104, 1264.6016) (-44.3065, 1261.2457) (-40.6857, 1252.3701) (-40.6857, 1247.0272) knots 0 0 0 1 2 2 2
  spline S165 degree 2 poles (-40.6857, 1247.0272) (-40.6857, 1241.5076) (-44.439, 1232.6762) (-48.104, 1229.4528) knots 0 0 0 1 2 2 2
  spline S166 degree 2 poles (-48.104, 1229.4528) (-51.7249, 1226.3176) (-62.3667, 1222.9617) (-69.0785, 1222.9617) knots 0 0 0 1 2 2 2
  spline S167 degree 2 poles (-69.0785, 1222.9617) (-75.9228, 1222.9617) (-86.3438, 1226.3618) (-90.0971, 1229.4969) knots 0 0 0 1 2 2 2
  spline S168 degree 2 poles (-90.0971, 1229.4969) (-93.718, 1232.6762) (-97.4713, 1241.5517) (-97.4713, 1247.0272) knots 0 0 0 1 2 2 2
  spline S169 degree 2 poles (-97.4713, 1247.0272) (-97.4713, 1252.5909) (-93.5855, 1261.5106) (-90.0971, 1264.6016) knots 0 0 0 1 2 2 2
  spline S170 degree 2 poles (-69.0785, 1263.586) (-74.4656, 1263.586) (-82.8113, 1261.2457) (-85.549, 1259.1261) knots 0 0 0 1 2 2 2
  spline S171 degree 2 poles (-85.549, 1259.1261) (-88.375, 1256.9624) (-91.2011, 1250.8688) (-91.2011, 1247.0713) knots 0 0 0 1 2 2 2
  spline S172 degree 2 poles (-91.2011, 1247.0713) (-91.2011, 1243.1414) (-88.4633, 1237.2243) (-85.549, 1234.9724) knots 0 0 0 1 2 2 2
  spline S173 degree 2 poles (-85.549, 1234.9724) (-82.7671, 1232.8087) (-74.3773, 1230.5125) (-69.0785, 1230.5125) knots 0 0 0 1 2 2 2
  spline S174 degree 2 poles (-69.0785, 1230.5125) (-58.3484, 1230.5125) (-46.9559, 1239.5205) (-46.9559, 1247.0713) knots 0 0 0 1 2 2 2
  spline S175 degree 2 poles (-46.9559, 1247.0713) (-46.9559, 1254.6221) (-58.3484, 1263.586) (-69.0785, 1263.586) knots 0 0 0 1 2 2 2
  spline S176 degree 2 poles (-40.6857, 1298.1166) (-40.6857, 1293.3035) (-43.2026, 1286.1501) (-45.7195, 1283.6332) knots 0 0 0 1 2 2 2
  spline S177 degree 2 poles (-45.7195, 1283.6332) (-48.5456, 1280.763) (-56.4938, 1278.4227) (-62.3225, 1278.4227) knots 0 0 0 1 2 2 2
  line L204 (-62.3225, 1278.4227) -> (-96.3232, 1278.4227)
  line L205 (-96.3232, 1278.4227) -> (-96.3232, 1285.6644)
  line L206 (-96.3232, 1285.6644) -> (-62.3225, 1285.6644)
  spline S178 degree 2 poles (-62.3225, 1285.6644) (-58.525, 1285.6644) (-53.4028, 1286.6358) (-51.3275, 1288.0047) knots 0 0 0 1 2 2 2
  spline S179 degree 2 poles (-51.3275, 1288.0047) (-49.1196, 1289.4619) (-46.8676, 1294.4957) (-46.8676, 1298.1166) knots 0 0 0 1 2 2 2
  spline S180 degree 2 poles (-46.8676, 1298.1166) (-46.8676, 1301.5167) (-49.1196, 1306.8155) (-51.3275, 1308.2727) knots 0 0 0 1 2 2 2
  spline S181 degree 2 poles (-51.3275, 1308.2727) (-53.4028, 1309.6415) (-58.4809, 1310.613) (-62.1459, 1310.613) knots 0 0 0 1 2 2 2
  line L207 (-62.1459, 1310.613) -> (-96.3232, 1310.613)
  line L208 (-96.3232, 1310.613) -> (-96.3232, 1317.8547)
  line L209 (-96.3232, 1317.8547) -> (-62.3225, 1317.8547)
  spline S182 degree 2 poles (-62.3225, 1317.8547) (-56.6263, 1317.8547) (-48.5014, 1315.5585) (-45.7195, 1312.6442) knots 0 0 0 1 2 2 2
  spline S183 degree 2 poles (-45.7195, 1312.6442) (-43.1584, 1310.0389) (-40.6857, 1303.1505) (-40.6857, 1298.1166) knots 0 0 0 1 2 2 2
  spline S184 degree 2 poles (-79.8969, 1362.6738) (-76.3644, 1362.6738) (-70.0058, 1360.1569) (-67.7979, 1357.9049) knots 0 0 0 1 2 2 2
  spline S185 degree 2 poles (-67.7979, 1357.9049) (-65.0161, 1355.0789) (-62.1459, 1347.4397) (-62.1459, 1341.611) knots 0 0 0 1 2 2 2
  line L210 (-62.1459, 1341.611) -> (-62.1459, 1335.4733)
  line L211 (-62.1459, 1335.4733) -> (-41.8337, 1335.4733)
  line L212 (-41.8337, 1335.4733) -> (-41.8337, 1328.2315)
  line L213 (-41.8337, 1328.2315) -> (-96.3232, 1328.2315)
  line L214 (-96.3232, 1328.2315) -> (-96.3232, 1341.9201)
  spline S186 degree 2 poles (-96.3232, 1341.9201) (-96.3232, 1346.7774) (-94.7336, 1353.5775) (-92.9232, 1356.1828) knots 0 0 0 1 2 2 2
  spline S187 degree 2 poles (-92.9232, 1356.1828) (-90.8478, 1359.2296) (-84.4451, 1362.6738) (-79.8969, 1362.6738) knots 0 0 0 1 2 2 2
  spline S188 degree 2 poles (-79.6761, 1355.123) (-82.5022, 1355.123) (-86.6529, 1353.1801) (-87.9776, 1351.1931) knots 0 0 0 1 2 2 2
  spline S189 degree 2 poles (-87.9776, 1351.1931) (-89.1257, 1349.471) (-90.053, 1344.8787) (-90.053, 1341.4786) knots 0 0 0 1 2 2 2
  line L215 (-90.053, 1341.4786) -> (-90.053, 1335.4733)
  line L216 (-90.053, 1335.4733) -> (-68.3278, 1335.4733)
  line L217 (-68.3278, 1335.4733) -> (-68.3278, 1340.4188)
  spline S190 degree 2 poles (-68.3278, 1340.4188) (-68.3278, 1344.8345) (-69.7408, 1350.2658) (-71.5954, 1352.0321) knots 0 0 0 1 2 2 2
  spline S191 degree 2 poles (-71.5954, 1352.0321) (-73.2292, 1353.6659) (-77.0709, 1355.123) (-79.6761, 1355.123) knots 0 0 0 1 2 2 2
  point P0 (0, 0)
  constraints: 4 other
extrude "Extrusion3" cut sketch "Sketch9" against normal blind 6.35
sketch "Sketch12" plane through (0, 22.225, 0) normal (0, 1, 0) x (1, 0, 0)
  line L0 (-271.6288, -542.9582) -> (-1290.4335, 1294.2578) construction
  line L1 (-1290.4335, 1294.2578) -> (-155.0341, 1923.8791) construction
  line L2 (-155.0341, 1923.8791) -> (863.7706, 86.6631) construction
  line L3 (863.7706, 86.6631) -> (-271.6288, -542.9582) construction
  point P0 (0, 0)
  constraints: 2 other
decal "Decal2"
body "Solid1"
